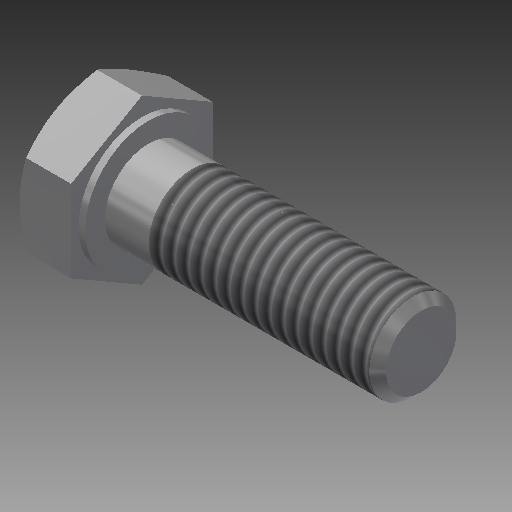
# Autodesk Inventor part: ISO 4017 - M8 x 25
Saved by Autodesk Inventor 2017 SP1 (Build 210196100, 196)
## iProperties
Library Location: C:\Program Files\Autodesk\Inventor 6\content
Library: local
SubLibrary: ISO
Family: 6
Member: 740
Member Major Revision: 1
Member Minor Revision: 1
Comments: To add or edit properties for Autodesk Inventor files, use iProperties.
Created: 2003-04-30
Part Number: ISO 4017 - M8 x 25
Vendor: Autodesk Inc.
Document SubType Name: Modeling
Designer: James M. Leake
Description: Hex-Head Bolt
Standard: ISO 4017 M8 x 25
Material: Steel, Mild
Density: 7.85 g/cm^3
Mass: 15.6919 g
Surface Area: 11.357 cm^2
Volume: 1.99897 cm^3
Appearance: Steel
Alert: To add or edit properties for Autodesk Inventor files, use iProperties.
Control State: 0
Master: False
Checked Out: False
Shininess: 64.0
Length Units: 11269
Angle Units: 11279
Time Units: 11290
Mass Units: 11283
Length Display Precision: 3
Angle Display Precision: 2
Compacted: True
EGR: 1
Density: 0.0
Volumn: 0.0
Area: 0.0
PropertySet Name: Model Information
Author: James M. Leake
Revision Number: 1
Autodesk Inventor part; units mm, degrees
ref_plane "YZ Plane" through (0, 0, 0) normal (1, 0, 0) x (0, 1, 0)
ref_plane "XZ Plane" through (0, 0, 0) normal (0, 1, 0) x (-1, 0, 0)
ref_plane "XY Plane" through (0, 0, 0) normal (0, 0, 1) x (1, 0, 0)
sketch "Sketch1" plane through (0, 0, 0) normal (0, 0, 1) x (1, 0, 0)
  line L0 (0, 5.815) -> (0, 4)
  line L1 (4, 4) -> (25, 4)
  line L2 (25, 4) -> (25, 0)
  line L3 (25, 0) -> (-0.6001, 0)
  line L4 (-3.0501, 0) -> (32.65, 0) projected
  line L5 (-0.6001, 0) -> (-0.6001, 5.815)
  line L6 (-0.6001, 5.815) -> (0, 5.815)
  line L7 (4, 4) -> (3.2331, 4)
  line L8 (3.2331, 4) -> (0, 4)
  line L9 (0, -0.344) -> (0, 4.472) projected
  dimension "d0" = 25
  dimension "d1" = 21
  dimension "d2" = 8
  dimension "d9" = 0.6001
  dimension "d10" = 11.63
  dimension "d13" = 0.7669
  dimension "d14" = 8
  constraints: 16 end point, 2 collinear, 2 perpendicular, 1 parallel
  measures "d0" distance between parallel lines of L2 L0
  measures "d1" distance from line of L1.start L2
  measures "d2" diameter of L1 L3
  measures "d9" distance between parallel lines of L5 L0
  measures "d10" diameter of L6 L3
  measures "d13" distance of L1.start L7.end
  measures "d14" diameter of L8 L3
revolve "Body" add sketch "Sketch1" angle 360 about axis through (25, 0, 0) along (-1, 0, 0)
sketch "Sketch2" plane through (-0.6001, 0, 0) normal (-1, 0, 0) x (0, 0, 1)
  line L0 (0, 7.5056) -> (6.5, 3.7528)
  line L1 (6.5, 3.7528) -> (6.5, -3.7528)
  line L2 (6.5, -3.7528) -> (0, -7.5056)
  line L3 (0, -7.5056) -> (-6.5, -3.7528)
  line L4 (-6.5, -3.7528) -> (-6.5, 3.7528)
  line L5 (-6.5, 3.7528) -> (0, 7.5056)
  point P0 (0, 0)
  point P1 (0, 0)
  dimension "d11" = 13
  constraints: 12 end point, 1 coincident, 1 vertical, 11 other
  measures "d11" distance between parallel lines of L4 L1
extrude "Head" add sketch "Sketch2" along normal blind 4.7
sketch "Sketch4" plane through (0, 0, 0) normal (0, 0, 1) x (1, 0, 0)
  line L0 (-5.3001, 6.5) -> (-5.3001, 7.5056)
  line L1 (-5.3001, 7.5056) -> (-4.7195, 7.5056)
  line L2 (-4.7195, 7.5056) -> (-5.3001, 6.5)
  line L3 (-3.8001, 0) -> (0.3999, 0) projected
  line L4 (-0.6001, 7.5056) -> (-5.3001, 7.5056) projected
  line L5 (-5.3001, 3.7528) -> (-5.3001, 7.5056) projected
  dimension "d5" = 30
  dimension "d19" = 13
  constraints: 6 end point, 2 collinear, 1 perpendicular, 1 vertical
  measures "d5" angle of L2 L0
  measures "d19" diameter of L0.start L3
revolve "Chamfer1" cut sketch "Sketch4" angle 360 about axis through (-10, 0, 0) along (1, 0, 0)
thread "Thread" size "M8x1.25" class "6g" standard "ISO Metric profile" length 21
chamfer "Chamfer2" distance 0.7668 distance2 0.7669 1 edges at (25, -4, 0) measured on face at (25, 0.998, -0.8842)
equation "\"d0\" = NLG"
equation "\"d1\" = GEL"
equation "\"d2\" = GD"
equation "\"d10\" = SD2"
equation "\"d14\" = BDM"
equation "\"d11\" = SW"
equation "\"d3\" = KOH - SD"
equation "\"d5\" = ANG1"
equation "\"d19\" = SW0"
equation "\"d15\" = GEL"
equation "\"d6\" = -0.5 * SPD + 0.5 * GD"
equation "\"NLG\" = 25"
equation "\"GD\" = NND"
equation "\"BDM\" = NND"
equation "\"KOH\" = 5.3"
equation "\"GEL\" = 21"
equation "\"SW\" = 13"
equation "\"SW0\" = SW"
equation "\"SPD\" = NND - 1.2269 * TPU"
equation "\"SD2\" = 11.63"
equation "\"SD\" = 0.6"
equation "\"ANG1\" = 30deg"
equation "\"GAL\" = 0.61345 * TPU"
equation "\"GUL\" = 0.61345 * TPU"
equation "\"RR\" = 0.4"
equation "\"d20\" = -NLG"
equation "\"TOA\" = 30deg"
equation "\"PTC\" = TPU"
equation "\"GD1\" = THREADDIA - 1.2269 * TPU"
equation "\"TPU\" = 1.25"
equation "\"THREADDIA\" = 8"
equation "\"SDH\" = SD2"
equation "\"E0\" = 15.015"
equation "\"NND\" = 8"
equation "\"SDHG\" = 4"
body "Solid1"
